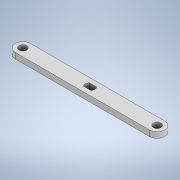
# Autodesk Inventor part: stuurarm motor
Saved by Autodesk Inventor 2022 (Build 260153000, 153)
## iProperties
Created: 2021-12-08
Part Number: stuurarm motor
Material: Generic
Document SubType Name: Modeling
Designer: keemi
Density: 1 g/cm^3
Appearance: Default
Author: keemi
Autodesk Inventor part; units mm, degrees
ref_plane "YZ Plane" through (0, 0, 0) normal (1, 0, 0) x (0, 1, 0)
ref_plane "XZ Plane" through (0, 0, 0) normal (0, 1, 0) x (-1, 0, 0)
ref_plane "XY Plane" through (0, 0, 0) normal (0, 0, 1) x (1, 0, 0)
sketch "Sketch1" plane through (0, 0, 0) normal (0, 1, 0) x (-1, 0, 0)
  line L0 (0, 0) -> (35, 0)
  line L1 (35, 0) -> (70, 0)
  circle A0 centre (70, 0) radius 2
  circle A1 centre (70, 0) radius 4
  circle A2 centre (0, 0) radius 4
  line L2 (0, 4) -> (70, 4)
  line L3 (0, -4) -> (70, -4)
  circle A3 centre (35, 0) radius 2.5
  line L4 (35, 0) -> (35, 1.5)
  line L5 (35, 1.5) -> (38.63, 1.5)
  line L6 (38.63, 1.5) -> (30.4744, 1.5)
  line L7 (30.4744, 1.5) -> (30.4744, -1.5)
  line L8 (30.4744, -1.5) -> (38.63, -1.5)
  line L9 (38.63, -1.5) -> (38.63, 1.5)
  circle A4 centre (0, 0) radius 2
  point P0 (37, 1.5)
  point P1 (37, -1.5)
  point P2 (33, -1.5)
  point P3 (33, 1.5)
  dimension "d1" = 35
  dimension "d2" = 35
  dimension "d3" = 4
  dimension "d4" = 8
  dimension "d5" = 8
  dimension "d6" = 5
  dimension "d7" = 1.5
  dimension "d8" = 3
  dimension "d9" = 4
  constraints: 20 end point, 5 centre point, 5 coincident, 4 point on circle, 3 horizontal, 3 tangent, 2 parallel, 1 perpendicular, 1 point on line, 1 vertical
  measures "d1" distance of L0.start L0.end
  measures "d2" distance of L0.end L1.end
  measures "d3" diameter of A0
  measures "d4" diameter of A1
  measures "d5" diameter of A2
  measures "d6" diameter of A3
  measures "d7" distance of L4.start L4.end
  measures "d8" distance of L7.end L6.end
  measures "d9" diameter of A4
extrude "Extrusion1" add sketch "Sketch1" along normal blind 3 contours A2 L2 A1 L1 L9 L5 A3 L6 L7 L0 | A2 | L0 L7 L8 A3 L9 L1 A1 L3 A2 | L7 L6 A3 L0 | L0 A3 L8 L7 | A1 | A3 L5 L6 | L8 A3 | A3 L5 L9 L1 | L1 L9 L8 A3
body "Solid1"
